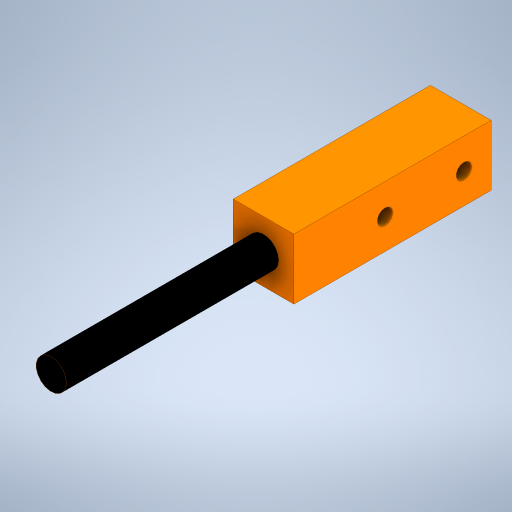
# Autodesk Inventor part: Base
Saved by Autodesk Inventor 2023.1 (Build 271208000, 208)
## iProperties
Created: 2022-11-06
Part Number: Base
Material: Generic
Document SubType Name: Modeling
Designer: shubh
Density: 1 g/cm^3
Appearance: Default(1)
Author: shubh
Autodesk Inventor part; units mm, degrees
ref_plane "YZ Plane" through (0, 0, 0) normal (1, 0, 0) x (0, 1, 0)
ref_plane "XZ Plane" through (0, 0, 0) normal (0, 1, 0) x (-1, 0, 0)
ref_plane "XY Plane" through (0, 0, 0) normal (0, 0, 1) x (1, 0, 0)
sketch "Sketch1" plane through (0, 0, 0) normal (1, 0, 0) x (0, 1, 0)
  line L0 (31.75, 38.1) -> (6.35, 38.1)
  line L1 (6.35, 38.1) -> (6.35, -19.05)
  line L2 (6.35, -19.05) -> (31.75, -19.05)
  circle A0 centre (19.0246, 25.4) radius 3.175
  line L3 (0, 0) -> (6.35, 0)
  line L4 (0, 14.2875) -> (0, -6.35)
  circle A1 centre (19.05, -7.62) radius 3.175
  line L5 (31.75, 38.1) -> (31.75, -25.4)
  point P0 (31.75, -19.05)
  dimension "d0" = 57.15
  dimension "d1" = 38.1
  dimension "d2" = 25.4
  dimension "d3" = 31.75
  dimension "d4" = 6.35
  dimension "d7" = 6.35
  dimension "d8" = 33.02
  constraints: 12 end point, 2 centre point, 2 horizontal, 2 vertical, 1 parallel, 1 perpendicular
  measures "d0" distance of L2.end L0.start
  measures "d1" vertical distance of L0.start L3.start
  measures "d2" distance of L0.start L0.end
  measures "d3" horizontal distance of L3.start L0.start
  measures "d4" diameter of A0
  measures "d7" diameter of A1
  measures "d8" distance of A1.centre A0.centre
extrude "Extrusion1" add sketch "Sketch1" along normal blind 25.4
sketch "Sketch2" plane through (0, 6.35, 38.1) normal (0, 0, 1) x (1, 0, 0)
  line L0 (0, 25.4) -> (25.4, 25.4) projected
  line L1 (25.4, 0) -> (0, 0)
  line L2 (0, 0) -> (0, 25.4)
  line L3 (0, 25.4) -> (25.4, 25.4)
  line L4 (25.4, 25.4) -> (25.4, 0)
  point P0 (0, -6.35)
  constraints: 8 end point, 2 parallel, 1 horizontal, 1 perpendicular
extrude "Extrusion2" add sketch "Sketch2" along normal blind 25.4
sketch "Sketch3" plane through (0, 6.35, 63.5) normal (0, 0, 1) x (1, 0, 0)
  circle A0 centre (12.7, 12.7) radius 6.35
  point P0 (0, -6.35)
  dimension "d18" = 12.7
  constraints: 1 centre point
  measures "d18" diameter of A0
extrude "Extrusion3" add sketch "Sketch3" along normal blind 88.9
body "Solid1"
